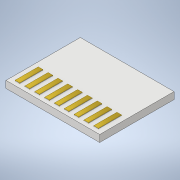
# Autodesk Inventor part: PCB
Saved by Autodesk Inventor 2020 (Build 240168000, 168)
## iProperties
Created: 2019-02-19
Part Number: PCB
Material: 일반
Document SubType Name: Modeling
Designer: Jeong Ji Hoon
Density: 1 g/cm^3
Appearance: 기본값
Author: Jeong Ji Hoon
Autodesk Inventor part; units mm, degrees
ref_plane "YZ Plane" through (0, 0, 0) normal (1, 0, 0) x (0, 1, 0)
ref_plane "XZ Plane" through (0, 0, 0) normal (0, 1, 0) x (-1, 0, 0)
ref_plane "XY Plane" through (0, 0, 0) normal (0, 0, 1) x (1, 0, 0)
sketch "스케치1" plane through (0, 0, 0) normal (0, 1, 0) x (-1, 0, 0)
  line L0 (0, 0) -> (12.1, 0)
  line L1 (12.1, 0) -> (12.1, -9.6)
  line L2 (12.1, -9.6) -> (0, -9.6)
  line L3 (0, -9.6) -> (0, 0)
  dimension "d0" = 12.1
  dimension "d1" = 9.6
  constraints: 8 end point, 2 parallel, 1 horizontal, 1 perpendicular
  measures "d0" distance of L1.end L2.end
  measures "d1" distance of L0.end L1.end
extrude "돌출1" add sketch "스케치1" along normal blind 0.9
sketch "스케치2" plane through (0, 0.9, 0) normal (0, 1, 0) x (1, 0, 0)
  line L0 (-11.43, 0.5) -> (-10.83, 0.5)
  line L1 (-10.83, 0.5) -> (-10.83, 3.5)
  line L2 (-10.83, 3.5) -> (-11.43, 3.5)
  line L3 (-11.43, 3.5) -> (-11.43, 0.5)
  line L4 (-12.1, 0) -> (0, 0) projected
  line L5 (-12.1, 9.6) -> (-12.1, 0) projected
  line L6 (-10.16, 0.5) -> (-9.56, 0.5)
  line L7 (-9.56, 0.5) -> (-9.56, 3.5)
  line L8 (-9.56, 3.5) -> (-10.16, 3.5)
  line L9 (-10.16, 3.5) -> (-10.16, 0.5)
  line L10 (-8.89, 0.5) -> (-8.29, 0.5)
  line L11 (-8.29, 0.5) -> (-8.29, 3.5)
  line L12 (-8.29, 3.5) -> (-8.89, 3.5)
  line L13 (-8.89, 3.5) -> (-8.89, 0.5)
  line L14 (-7.62, 0.5) -> (-7.02, 0.5)
  line L15 (-7.02, 0.5) -> (-7.02, 3.5)
  line L16 (-7.02, 3.5) -> (-7.62, 3.5)
  line L17 (-7.62, 3.5) -> (-7.62, 0.5)
  line L18 (-6.35, 0.5) -> (-5.75, 0.5)
  line L19 (-5.75, 0.5) -> (-5.75, 3.5)
  line L20 (-5.75, 3.5) -> (-6.35, 3.5)
  line L21 (-6.35, 3.5) -> (-6.35, 0.5)
  line L22 (-5.08, 0.5) -> (-4.48, 0.5)
  line L23 (-4.48, 0.5) -> (-4.48, 3.5)
  line L24 (-4.48, 3.5) -> (-5.08, 3.5)
  line L25 (-5.08, 3.5) -> (-5.08, 0.5)
  line L26 (-3.81, 0.5) -> (-3.21, 0.5)
  line L27 (-3.21, 0.5) -> (-3.21, 3.5)
  line L28 (-3.21, 3.5) -> (-3.81, 3.5)
  line L29 (-3.81, 3.5) -> (-3.81, 0.5)
  line L30 (-2.54, 0.5) -> (-1.94, 0.5)
  line L31 (-1.94, 0.5) -> (-1.94, 3.5)
  line L32 (-1.94, 3.5) -> (-2.54, 3.5)
  line L33 (-2.54, 3.5) -> (-2.54, 0.5)
  line L34 (-1.27, 0.5) -> (-0.67, 0.5)
  line L35 (-0.67, 0.5) -> (-0.67, 3.5)
  line L36 (-0.67, 3.5) -> (-1.27, 3.5)
  line L37 (-1.27, 3.5) -> (-1.27, 0.5)
  line L38 (0, 0) -> (0, 9.6) projected
  point P0 (-6.05, 0.5)
  point P1 (-6.05, 0)
  dimension "d4" = 0.6
  dimension "d5" = 3
  dimension "d6" = 0.5
  dimension "d10" = 1.27
  dimension "d15" = 0.67
  constraints: 72 end point, 2 horizontal, 2 midpoint, 2 parallel, 1 perpendicular, 1 vertical alignment, 64 other
  measures "d4" distance of L2.end L1.end
  measures "d5" distance of L1.end L0.end
  measures "d6" distance between parallel lines of L4 L0
  measures "d10" distance of L0.start L6.start
  measures "d15" distance between parallel lines of L35 L38
extrude "돌출2" add sketch "스케치2" along normal blind 0.1 and the other way blind 1 separate body
